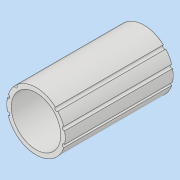
# Autodesk Inventor part: pistonTank
Saved by Autodesk Inventor 2017 (Build 210142000, 142)
## iProperties
Created: 2016-11-20
Part Number: pistonTank
Material: UHMW, White
Document SubType Name: Modeling
Designer: techn
Density: 0.94 g/cm^3
Appearance: Smooth - White
Mass: 207.673 g
Surface Area: 792.921 cm^2
Volume: 220.929 cm^3
Author: techn
Autodesk Inventor part; units mm, degrees
ref_plane "YZ Plane" through (0, 0, 0) normal (1, 0, 0) x (0, 1, 0)
ref_plane "XZ Plane" through (0, 0, 0) normal (0, 1, 0) x (-1, 0, 0)
ref_plane "XY Plane" through (0, 0, 0) normal (0, 0, 1) x (1, 0, 0)
sketch "Sketch1" plane through (0, 0, 0) normal (0, 0, 1) x (1, 0, 0)
  circle A0 centre (0, 0) radius 41.275
  circle A1 centre (0, 0) radius 34.925
  dimension "d0" = 82.55
  dimension "d1" = 69.85
  constraints: 2 centre point, 2 coincident
  measures "d0" diameter of A0
  measures "d1" diameter of A1
extrude "Extrusion1" add sketch "Sketch1" along normal blind 152.4
sketch "Sketch3" plane through (0, 0, 152.4) normal (0, 0, 1) x (1, 0, 0)
  line L0 (0, 0) -> (39.3779, 10.5513)
  line L1 (0, 0) -> (40.767, 0) construction
  circle A0 centre (39.3779, 10.5513) radius 2.4447
  line L2 (0, 0) -> (0, 11.1299)
  circle A1 centre (39.3779, -10.5513) radius 2.4447
  circle A2 centre (-39.3779, 10.5513) radius 2.4447
  circle A3 centre (-39.3779, -10.5513) radius 2.4447
  circle A4 centre (28.8266, 28.8266) radius 2.4447
  line L3 (28.8266, 28.8266) -> (0, 0)
  circle A5 centre (-28.8266, 28.8266) radius 2.4447
  dimension "d10" = 40.767
  dimension "d11" = 15
  dimension "d12" = 4.8895
  dimension "d15" = 45
  dimension "d16" = 4.8895
  dimension "d17" = 40.767
  constraints: 8 end point, 6 centre point, 4 symmetric about line, 1 coincident, 1 equal length, 1 horizontal, 1 vertical, 4 other
  measures "d10" distance of L0.start L0.end
  measures "d11" angle of L1 L0
  measures "d12" diameter of A0
  measures "d15" angle of L1 L3
  measures "d16" diameter of A4
  measures "d17" distance of L3.start L0.start
extrude "Extrusion3" cut sketch "Sketch3" against normal through all contours A0 | A1 | A2 | A3
extrude "Extrusion4" cut sketch "Sketch3" against normal through all contours A4 | A5
equation "\"d16\" = d12"
equation "\"d17\" = d10"
body "Solid1"
